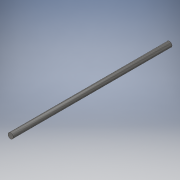
# Autodesk Inventor part: Hopper M6 rod
Saved by Autodesk Inventor 2018 (Build 220112000, 112)
## iProperties
Created: 2013-10-16
Part Number: Hopper M6 rod
Material: Steel, Carbon
Document SubType Name: Modeling
Designer: Gabriel Smolnycki
Mass: 39.9516 g
Surface Area: 34.4947 cm^2
Volume: 5.08938 cm^3
Density: 7.85 g/cm^3
Appearance: Semi-Polished
Sending System: SolidWorks 2017
Last Author: Gabriel Smolnycki
Last Saved: 2017-09-14
Author: Gabriel Smolnycki
Autodesk Inventor part; units mm, degrees
ref_plane "YZ Plane" through (0, 0, 0) normal (1, 0, 0) x (0, 1, 0)
ref_plane "XZ Plane" through (0, 0, 0) normal (0, 1, 0) x (-1, 0, 0)
ref_plane "Work Plane1" through (0, 0, -90) normal (0, 0, 1) x (1, 0, 0)
sketch "Sketch1" plane through (0, 0, -90) normal (0, 0, 1) x (1, 0, 0)
  circle A0 centre (0, 0) radius 3
  constraints: 1 centre point
extrude "Extrusion1" add sketch "Sketch1" along normal blind 180
thread "Thread1" size "M6x1" class "6g" standard "ISO Metric profile" full length
body "Solid3"
